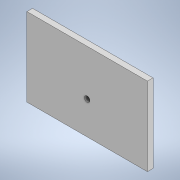
# Autodesk Inventor part: SoporteBaseElevacion
Saved by Autodesk Inventor 2021 (Build 250183000, 183)
## iProperties
Created: 2021-04-17
Part Number: SoporteBaseElevacion
Material: Generic
Document SubType Name: Modeling
Designer: GABRIEL LOL
Density: 1 g/cm^3
Appearance: Default
Author: GABRIEL LOL
Autodesk Inventor part; units mm, degrees
ref_plane "YZ Plane" through (0, 0, 0) normal (1, 0, 0) x (0, 1, 0)
ref_plane "XZ Plane" through (0, 0, 0) normal (0, 1, 0) x (-1, 0, 0)
ref_plane "XY Plane" through (0, 0, 0) normal (0, 0, 1) x (1, 0, 0)
sketch "Sketch1" plane through (0, 0, 0) normal (0, 0, 1) x (1, 0, 0)
  line L0 (-215, 140) -> (215, 140)
  line L1 (215, 140) -> (215, -140)
  line L2 (215, -140) -> (-215, -140)
  line L3 (-215, -140) -> (-215, 140)
  line L4 (-215, 140) -> (215, -140) construction
  line L5 (215, 140) -> (-215, -140) construction
  line L6 (0, 0) -> (0, -23) construction
  circle A0 centre (0, -23) radius 10
  dimension "d0" = 430
  dimension "d1" = 280
  dimension "d2" = 23
  dimension "d3" = 20
  constraints: 14 end point, 2 midpoint, 2 parallel, 1 centre point, 1 coincident, 1 horizontal, 1 perpendicular, 1 vertical
  measures "d0" distance of L1.end L2.end
  measures "d1" distance of L0.end L1.end
  measures "d2" distance of L6.start L6.end
  measures "d3" diameter of A0
extrude "Extrusion1" add sketch "Sketch1" along normal blind 20
sketch "Sketch2" plane through (0, 0, 0) normal (0, 0, -1) x (-1, 0, 0)
  line L0 (215, -140) -> (-215, -140) projected
  line L1 (215, 140) -> (215, -140) projected
  line L2 (-215, 140) -> (215, 140) projected
  line L3 (-215, -140) -> (-215, 140) projected
  circle A0 centre (0, -23) radius 10 projected
  line L4 (213, 138) -> (213, -138)
  line L5 (213, -138) -> (-213, -138)
  line L6 (-213, -138) -> (-213, 138)
  line L7 (-213, 138) -> (213, 138)
  point P0 (0, 0)
  dimension "d6" = 2
  constraints: 8 end point, 3 other
  measures "d6" distance between parallel lines of L2 L7
emboss "Emboss1" sketch "Sketch2" operation cut depth 1 direction (0, 0, 1) contours L4 L5 L6 L7
body "Solid1"
